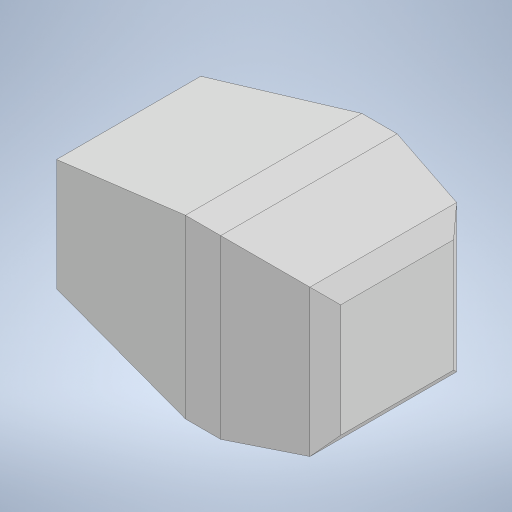
# Autodesk Inventor part: Scorpion Body
Saved by Autodesk Inventor 2024 (Build 280153000, 153)
## iProperties
Created: 2023-05-22
Part Number: Scorpion Body
Material: Generic
Document SubType Name: Modeling
Designer: vilas
Density: 1 g/cm^3
Appearance: Default
Author: vilas
Autodesk Inventor part; units mm, degrees
ref_plane "YZ Plane" through (0, 0, 0) normal (1, 0, 0) x (0, 1, 0)
ref_plane "XZ Plane" through (0, 0, 0) normal (0, 1, 0) x (-1, 0, 0)
ref_plane "XY Plane" through (0, 0, 0) normal (0, 0, 1) x (1, 0, 0)
sketch "Sketch1" plane through (0, 0, 0) normal (0, 0, 1) x (1, 0, 0)
  line L0 (0, 0) -> (400, 0)
  line L1 (400, 0) -> (400, 250)
  line L2 (400, 250) -> (0, 250)
  line L3 (0, 250) -> (0, 0)
  dimension "d0" = 400
  dimension "d1" = 250
  constraints: 8 end point, 2 horizontal, 2 parallel, 1 perpendicular, 1 vertical
  measures "d0" distance of L2.end L1.end
  measures "d1" distance of L1.end L0.end
extrude "Extrusion1" add sketch "Sketch1" along normal mid plane 250
sketch "Sketch2" plane through (0, 0, 0) normal (0, 0, 1) x (1, 0, 0)
  line L0 (400, 0) -> (400, 250) projected
  line L1 (400, 225) -> (275, 250)
  line L2 (400, 250) -> (0, 250) projected
  line L3 (275, 250) -> (400, 250)
  line L4 (400, 225) -> (400, 250)
  line L5 (400, 25) -> (275, 0)
  line L6 (0, 0) -> (400, 0) projected
  line L7 (225, 250) -> (0, 200)
  line L8 (0, 250) -> (0, 0) projected
  line L9 (225, 0) -> (0, 50)
  line L10 (400, 25) -> (400, 0)
  line L11 (275, 0) -> (400, 0)
  line L12 (225, 0) -> (0, 0)
  line L13 (0, 0) -> (0, 50)
  line L14 (0, 200) -> (0, 250)
  line L15 (225, 250) -> (0, 250)
  dimension "d4" = 25
  dimension "d5" = 125
  dimension "d6" = 25
  dimension "d7" = 125
  dimension "d8" = 50
  dimension "d9" = 50
  dimension "d10" = 50
  dimension "d11" = 50
  constraints: 24 end point, 8 point on line, 7 collinear, 1 perpendicular
  measures "d4" distance of L1.start L0.end
  measures "d5" distance of L1.end L0.end
  measures "d6" distance of L5.start L0.start
  measures "d7" distance of L5.end L0.start
  measures "d8" distance of L7.start L1.end
  measures "d9" distance of L9.start L5.end
  measures "d10" distance of L7.end L2.end
  measures "d11" distance of L6.start L9.end
extrude "Extrusion2" cut sketch "Sketch2" along normal through all both and the other way through all contours L6 L5 L0 | L1 L2 L0 | L6 L8 L9 | L7 L8 L2
sketch "Sketch3" plane through (0, 0, 0) normal (0, 1, 0) x (-1, 0, 0)
  line L0 (-275, -125) -> (-400, -125)
  line L1 (-400, -125) -> (-400, -100)
  line L2 (-400, -100) -> (-275, -125)
  line L3 (-275, 125) -> (-400, 125)
  line L4 (-400, 125) -> (-400, 100)
  line L5 (-275, 125) -> (-400, 100)
  line L6 (0, 0) -> (-400, 0) construction
  line L7 (0, 0) -> (0, 125) construction
  line L8 (0, 0) -> (0, -125) construction
  dimension "d28" = 25
  dimension "d29" = 25
  dimension "d32" = 400
  dimension "d33" = 100
  dimension "d34" = 100
  dimension "d35" = 125
  dimension "d36" = 125
  dimension "d37" = 125
  dimension "d38" = 125
  dimension "d39" = 400
  dimension "d40" = 400
  constraints: 18 end point, 3 horizontal, 2 perpendicular, 2 vertical
  measures "d28" distance of L0.end L1.end
  measures "d29" distance of L3.end L4.end
  measures "d32" distance of L6.start L6.end
  measures "d33" distance from line of L6 L4.end
  measures "d34" distance from line of L1.end L6
  measures "d35" distance from line of L4 L3.start
  measures "d36" distance from line of L1 L0.start
  measures "d37" distance of L6.start L7.end
  measures "d38" distance of L6.start L8.end
  measures "d39" distance from line of L4 L7.end
  measures "d40" distance between parallel lines of L1 L8
extrude "Extrusion3" cut sketch "Sketch3" along normal through all
sketch "Sketch4" plane through (0, 0, 0) normal (0, 1, 0) x (-1, 0, 0)
  line L0 (0, -125) -> (-400, -125) projected
  line L1 (-225, -125) -> (0, -125)
  line L2 (0, -125) -> (0, -100)
  line L3 (0, -100) -> (-225, -125)
  line L4 (-225, 125) -> (0, 125) projected
  line L5 (-225, 125) -> (0, 125)
  line L6 (0, 125) -> (0, 100)
  line L7 (0, 100) -> (-225, 125)
  point P0 (0, 0)
  point P1 (-275, -125)
  dimension "d18" = 25
  dimension "d19" = 25
  constraints: 12 end point, 2 perpendicular, 1 horizontal
  measures "d18" distance of L4.end L6.end
  measures "d19" distance of L1.end L2.end
extrude "Extrusion4" cut sketch "Sketch4" along normal through all
chamfer "Chamfer1" distance 20 angle 45 4 edges at (0, 125, -100) (0, 125, 100) (0, 200, 0) (0, 50, 0)
chamfer "Chamfer2" distance 20 angle 45 4 edges at (400, 225, 0) (400, 125, -100) (400, 125, 100) (400, 25, 0)
body "Solid1"
